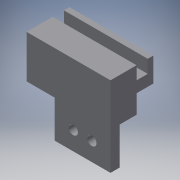
# Autodesk Inventor part: suporte p trilho
Saved by Autodesk Inventor 2018 (Build 220112000, 112)
## iProperties
Created: 2018-05-30
Part Number: suporte p trilho
Material: Genérico
Document SubType Name: Modeling
Designer: Ernandes
Density: 1 g/cm^3
Appearance: Padrão
Author: Ernandes
Autodesk Inventor part; units mm, degrees
ref_plane "YZ Plane" through (0, 0, 0) normal (1, 0, 0) x (0, 1, 0)
ref_plane "XZ Plane" through (0, 0, 0) normal (0, 1, 0) x (-1, 0, 0)
ref_plane "XY Plane" through (0, 0, 0) normal (0, 0, 1) x (1, 0, 0)
sketch "Esboço1" plane through (0, 0, 0) normal (0, 1, 0) x (-1, 0, 0)
  line L0 (0, 0) -> (0, -20)
  line L1 (0, -20) -> (30, -20)
  line L2 (30, -20) -> (30, 0)
  line L3 (30, 0) -> (0, 0)
  circle A0 centre (15, -10) radius 2.5
  dimension "d0" = 20
  dimension "d1" = 30
  dimension "d2" = 5
  constraints: 8 end point, 3 perpendicular, 1 centre point, 1 vertical
  measures "d0" distance of L0.start L0.end
  measures "d1" distance of L0.end L1.end
  measures "d2" diameter of A0
extrude "Extrusão1" add sketch "Esboço1" along normal blind 5
sketch "Esboço2" plane through (0, 0, 0) normal (0, -1, 0) x (1, 0, 0)
  line L0 (0, 0) -> (0, 23)
  line L1 (0, 23) -> (-45, 23)
  line L2 (-45, 23) -> (-45, 0)
  line L3 (-45, 0) -> (0, 0)
  dimension "d5" = 23
  dimension "d6" = 45
  constraints: 8 end point, 3 perpendicular, 1 vertical
  measures "d5" distance of L0.start L0.end
  measures "d6" distance of L0.end L1.end
extrude "Extrusão2" add sketch "Esboço2" against normal blind 14
sketch "Esboço3" plane through (0, 14, 0) normal (0, 1, 0) x (1, 0, 0)
  line L0 (0, -23) -> (0, 20) projected
  line L1 (0, -23) -> (0, -16)
  line L2 (0, -16) -> (-45, -16)
  line L3 (-45, 0) -> (-45, -23) projected
  line L4 (-45, -16) -> (-45, -10)
  line L5 (-45, -10) -> (0, -10)
  line L6 (0, -10) -> (0, -16)
  point P0 (0, 0)
  dimension "d9" = 7
  dimension "d10" = 6
  constraints: 10 end point, 4 perpendicular, 3 point on line
  measures "d9" distance of L0.start L1.end
  measures "d10" distance of L2.end L4.end
extrude "Extrusão3" add sketch "Esboço3" along normal blind 6
sketch "Esboço4" plane through (0, 20, 0) normal (0, 1, 0) x (1, 0, 0)
  line L0 (-45, -10) -> (0, -10) projected
  line L1 (-45, -23) -> (-45, 0) projected
  line L2 (-45, -10) -> (-45, -23)
  line L3 (-45, -23) -> (0, -23) projected
  line L4 (-45, -23) -> (0, -23)
  line L5 (0, -16) -> (0, -10) projected
  line L6 (0, -23) -> (0, -10)
  line L7 (0, -10) -> (-45, -10)
  point P0 (0, 0)
  constraints: 8 end point, 2 collinear, 2 perpendicular
extrude "Extrusão4" add sketch "Esboço4" along normal blind 3
sketch "Esboço5" plane through (-45, 0, 0) normal (-1, 0, 0) x (0, 0, 1)
  line L0 (10, 14) -> (12.7, 14)
  line L1 (12.7, 14) -> (12.7, 9.5)
  line L2 (12.7, 9.5) -> (10, 9.5)
  line L3 (10, 14) -> (10, 23) projected
  line L4 (10, 9.5) -> (10, 14)
  point P0 (0, 0)
  dimension "d15" = 2.7
  dimension "d16" = 4.5
  constraints: 8 end point, 3 perpendicular, 1 horizontal
  measures "d15" distance of L0.start L0.end
  measures "d16" distance of L0.end L1.end
extrude "Extrusão5" add sketch "Esboço5" along normal blind 10
offset faces "Tamanho1" outward -10 faces at (-55, 12.5, 10.9)
sketch "Esboço6" plane through (0, 5, 0) normal (0, 1, 0) x (1, 0, 0)
  line L0 (0, -23) -> (0, 20) projected
  line L1 (0, 20) -> (-15, 20)
  line L2 (0, 20) -> (-30, 20) projected
  line L3 (-15, 20) -> (-15, 10)
  circle A0 centre (-15, 10) radius 2.5
  point P0 (0, 0)
  dimension "d20" = 10
  constraints: 4 end point, 1 centre point, 1 coincident, 1 midpoint, 1 perpendicular
  measures "d20" distance of L1.end L3.end
extrude "Extrusão6" add sketch "Esboço6" against normal blind 5
sketch "Esboço7" plane through (0, 5, 0) normal (0, 1, 0) x (1, 0, 0)
  line L0 (0, 20) -> (-30, 20) projected
  line L1 (0, 20) -> (-10, 20)
  line L2 (-10, 20) -> (-20, 20)
  line L3 (-20, 20) -> (-20, 10)
  line L4 (-10, 20) -> (-10, 10)
  circle A0 centre (-10, 10) radius 2.5
  circle A1 centre (-20, 10) radius 2.5
  point P0 (0, 0)
  dimension "d23" = 10
  dimension "d24" = 10
  dimension "d25" = 10
  dimension "d26" = 5
  constraints: 8 end point, 2 centre point, 2 coincident, 2 point on line, 1 perpendicular, 1 vertical
  measures "d23" distance of L0.start L1.end
  measures "d24" distance of L1.end L2.end
  measures "d25" distance of L2.end L3.end
  measures "d26" diameter of A0
extrude "Extrusão7" cut sketch "Esboço7" against normal blind 5
